Autodesk Fusion 360 part; units mm, degrees
(part 2 of 8)
  spline S4 degree 5 poles (18.7513, 10.1044) (18.7514, 10.1045) (18.7517, 10.1046) (18.7521, 10.1049) (18.7528, 10.1053) (18.7538, 10.1058) (18.755, 10.1065) (18.7564, 10.1073) (18.7579, 10.1081) (18.7595, 10.1091) (18.7613, 10.1102) (18.7633, 10.1113) (18.7654, 10.1125) (18.7676, 10.1138) (18.7699, 10.1153) (18.7724, 10.1168) (18.775, 10.1183) (18.7778, 10.12) (18.7807, 10.1218) (18.7836, 10.1236) (18.7868, 10.1256) (18.79, 10.1276) (18.7933, 10.1297) (18.7968, 10.1319) (18.8003, 10.1341) (18.804, 10.1365) (18.8078, 10.1389) (18.8117, 10.1414) (18.8157, 10.144) (18.8198, 10.1467) (18.824, 10.1495) (18.8282, 10.1523) (18.8326, 10.1553) (18.8371, 10.1583) (18.8417, 10.1613) (18.8463, 10.1645) (18.8511, 10.1677) (18.8559, 10.1711) (18.8608, 10.1745) (18.8658, 10.1779) (18.8709, 10.1815) (18.8761, 10.1851) (18.8814, 10.1888) (18.8867, 10.1926) (18.8921, 10.1965) (18.8976, 10.2004) (18.9032, 10.2044) (18.9088, 10.2085) (18.9145, 10.2127) (18.9203, 10.2169) (18.9262, 10.2212) (18.9321, 10.2256) (18.9381, 10.23) (18.9442, 10.2346) (18.9503, 10.2392) (18.9565, 10.2439) (18.9628, 10.2486) (18.9691, 10.2534) (18.9755, 10.2583) (18.982, 10.2633) (18.9885, 10.2683) (18.9951, 10.2735) (19.0017, 10.2786) (19.0085, 10.2839) (19.0152, 10.2892) (19.022, 10.2946) (19.0289, 10.3001) (19.0358, 10.3056) (19.0428, 10.3112) (19.0498, 10.3169) (19.0569, 10.3227) (19.0641, 10.3285) (19.0713, 10.3344) (19.0785, 10.3403) (19.0858, 10.3464) (19.0932, 10.3525) (19.1006, 10.3586) (19.108, 10.3649) (19.1155, 10.3712) (19.123, 10.3775) (19.1306, 10.384) (19.1382, 10.3905) (19.1459, 10.397) (19.1536, 10.4037) (19.1614, 10.4104) (19.1692, 10.4172) (19.177, 10.424) (19.1849, 10.4309) (19.1929, 10.4379) (19.2008, 10.4449) (19.2088, 10.452) (19.2169, 10.4592) (19.225, 10.4665) (19.2331, 10.4738) (19.2413, 10.4811) (19.2495, 10.4886) (19.2577, 10.4961) (19.266, 10.5036) (19.2743, 10.5113) (19.2826, 10.519) (19.291, 10.5267) (19.2994, 10.5346) (19.3079, 10.5425) (19.3163, 10.5504) (19.3249, 10.5584) (19.3334, 10.5665) (19.342, 10.5747) (19.3506, 10.5829) (19.3592, 10.5912) (19.3679, 10.5995) (19.3766, 10.6079) (19.3853, 10.6164) (19.3941, 10.6249) (19.4028, 10.6335) (19.4116, 10.6421) (19.4205, 10.6509) (19.4293, 10.6596) (19.4382, 10.6685) (19.4472, 10.6774) (19.4561, 10.6864) (19.4651, 10.6954) (19.4741, 10.7045) (19.4831, 10.7136) (19.4921, 10.7229) (19.5012, 10.7321) (19.5103, 10.7415) (19.5194, 10.7509) (19.5285, 10.7603) (19.5377, 10.7698) (19.5469, 10.7794) (19.5561, 10.7891) (19.5653, 10.7988) (19.5745, 10.8085) (19.5838, 10.8184) (19.5931, 10.8282) (19.6024, 10.8382) (19.6117, 10.8482) (19.621, 10.8583) (19.6304, 10.8684) (19.6398, 10.8786) (19.6492, 10.8888) (19.6586, 10.8991) (19.668, 10.9095) (19.6775, 10.9199) (19.6869, 10.9304) (19.6964, 10.9409) (19.7059, 10.9515) (19.7154, 10.9622) (19.725, 10.9729) (19.7345, 10.9837) (19.7441, 10.9945) (19.7536, 11.0054) (19.7632, 11.0164) (19.7728, 11.0274) (19.7824, 11.0384) (19.7921, 11.0496) (19.8017, 11.0607) (19.8113, 11.072) (19.821, 11.0833) (19.8307, 11.0946) (19.8404, 11.1061) (19.8501, 11.1175) (19.8598, 11.1291) (19.8695, 11.1406) (19.8792, 11.1523) (19.889, 11.164) (19.8987, 11.1757) (19.9085, 11.1875) (19.9183, 11.1994) (19.9281, 11.2113) (19.9379, 11.2233) (19.9477, 11.2354) (19.9575, 11.2475) (19.9673, 11.2596) (19.9771, 11.2718) (19.9869, 11.2841) (19.9968, 11.2964) (20.0066, 11.3088) (20.0165, 11.3212) (20.0263, 11.3337) (20.0362, 11.3462) (20.0461, 11.3588) (20.056, 11.3715) (20.0659, 11.3842) (20.0757, 11.3969) (20.0856, 11.4097) (20.0955, 11.4226) (20.1054, 11.4355) (20.1154, 11.4485) (20.1253, 11.4615) (20.1352, 11.4746) (20.1451, 11.4878) (20.155, 11.501) (20.165, 11.5142) (20.1749, 11.5275) (20.1848, 11.5409) (20.1948, 11.5543) (20.2047, 11.5677) (20.2147, 11.5813) (20.2246, 11.5948) (20.2346, 11.6085) (20.2445, 11.6221) (20.2545, 11.6359) (20.2644, 11.6497) (20.2744, 11.6635) (20.2843, 11.6774) (20.2943, 11.6913) (20.3042, 11.7053) (20.3142, 11.7194) (20.3242, 11.7335) (20.3341, 11.7476) (20.3441, 11.7618) (20.354, 11.7761) (20.364, 11.7904) (20.3739, 11.8048) (20.3839, 11.8192) (20.3938, 11.8336) (20.4038, 11.8482) (20.4137, 11.8627) (20.4237, 11.8773) (20.4336, 11.892) (20.4436, 11.9067) (20.4535, 11.9215) (20.4634, 11.9363) (20.4734, 11.9512) (20.4833, 11.9661) (20.4932, 11.9811) (20.5032, 11.9962) (20.5131, 12.0112) (20.523, 12.0264) (20.5329, 12.0416) (20.5428, 12.0568) (20.5527, 12.0721) (20.5626, 12.0874) (20.5725, 12.1028) (20.5824, 12.1182) (20.5923, 12.1337) (20.6022, 12.1492) (20.6121, 12.1648) (20.6219, 12.1805) (20.6318, 12.1961) (20.6397, 12.2087) (20.6456, 12.2182) (20.6495, 12.2245) (20.6515, 12.2277) knots 0 0 0 0 0 0 0.00416667 0.00833333 0.0125 0.01666667 0.02083333 0.025 0.02916667 0.03333333 0.0375 0.04166667 0.04583333 0.05 0.05416667 0.05833333 0.0625 0.06666667 0.07083333 0.075 0.07916667 0.08333333 0.0875 0.09166667 0.09583333 0.1 0.10416667 0.10833333 0.1125 0.11666667 0.12083333 0.125 0.12916667 0.13333333 0.1375 0.14166667 0.14583333 0.15 0.15416667 0.15833333 0.1625 0.16666667 0.17083333 0.175 0.17916667 0.18333333 0.1875 0.19166667 0.19583333 0.2 0.20416667 0.20833333 0.2125 0.21666667 0.22083333 0.225 0.22916667 0.23333333 0.2375 0.24166667 0.24583333 0.25 0.25416667 0.25833333 0.2625 0.26666667 0.27083333 0.275 0.27916667 0.28333333 0.2875 0.29166667 0.29583333 0.3 0.30416667 0.30833333 0.3125 0.31666667 0.32083333 0.325 0.32916667 0.33333333 0.3375 0.34166667 0.34583333 0.35 0.35416667 0.35833333 0.3625 0.36666667 0.37083333 0.375 0.37916667 0.38333333 0.3875 0.39166667 0.39583333 0.4 0.40416667 0.40833333 0.4125 0.41666667 0.42083333 0.425 0.42916667 0.43333333 0.4375 0.44166667 0.44583333 0.45 0.45416667 0.45833333 0.4625 0.46666667 0.47083333 0.475 0.47916667 0.48333333 0.4875 0.49166667 0.49583333 0.5 0.50416667 0.50833333 0.5125 0.51666667 0.52083333 0.525 0.52916667 0.53333333 0.5375 0.54166667 0.54583333 0.55 0.55416667 0.55833333 0.5625 0.56666667 0.57083333 0.575 0.57916667 0.58333333 0.5875 0.59166667 0.59583333 0.6 0.60416667 0.60833333 0.6125 0.61666667 0.62083333 0.625 0.62916667 0.63333333 0.6375 0.64166667 0.64583333 0.65 0.65416667 0.65833333 0.6625 0.66666667 0.67083333 0.675 0.67916667 0.68333333 0.6875 0.69166667 0.69583333 0.7 0.70416667 0.70833333 0.7125 0.71666667 0.72083333 0.725 0.72916667 0.73333333 0.7375 0.74166667 0.74583333 0.75 0.75416667 0.75833333 0.7625 0.76666667 0.77083333 0.775 0.77916667 0.78333333 0.7875 0.79166667 0.79583333 0.8 0.80416667 0.80833333 0.8125 0.81666667 0.82083333 0.825 0.82916667 0.83333333 0.8375 0.84166667 0.84583333 0.85 0.85416667 0.85833333 0.8625 0.86666667 0.87083333 0.875 0.87916667 0.88333333 0.8875 0.89166667 0.89583333 0.9 0.90416667 0.90833333 0.9125 0.91666667 0.92083333 0.925 0.92916667 0.93333333 0.9375 0.94166667 0.94583333 0.95 0.95416667 0.95833333 0.9625 0.96666667 0.97083333 0.975 0.97916667 0.98333333 0.9875 0.99166667 0.99583333 1 1 1 1 1 1
  arc A5 (20.6515, 12.2277) -> (19.7016, 13.7057) centre (0, 0) ccw
  spline S5 degree 5 poles (19.7016, 13.7057) (19.6979, 13.7052) (19.6905, 13.7043) (19.6795, 13.7028) (19.6647, 13.7009) (19.6464, 13.6984) (19.6281, 13.6959) (19.6098, 13.6934) (19.5916, 13.6909) (19.5734, 13.6883) (19.5552, 13.6857) (19.5371, 13.6831) (19.519, 13.6805) (19.501, 13.6778) (19.4831, 13.6752) (19.4651, 13.6724) (19.4472, 13.6697) (19.4294, 13.6669) (19.4116, 13.6642) (19.3939, 13.6614) (19.3762, 13.6585) (19.3585, 13.6557) (19.3409, 13.6528) (19.3233, 13.6499) (19.3058, 13.647) (19.2883, 13.644) (19.2709, 13.641) (19.2535, 13.638) (19.2362, 13.635) (19.2189, 13.632) (19.2016, 13.6289) (19.1844, 13.6258) (19.1673, 13.6227) (19.1502, 13.6196) (19.1331, 13.6164) (19.1161, 13.6132) (19.0991, 13.61) (19.0822, 13.6068) (19.0654, 13.6036) (19.0485, 13.6003) (19.0318, 13.597) (19.015, 13.5937) (18.9984, 13.5904) (18.9817, 13.5871) (18.9652, 13.5837) (18.9486, 13.5803) (18.9322, 13.5769) (18.9157, 13.5735) (18.8994, 13.57) (18.883, 13.5665) (18.8668, 13.563) (18.8505, 13.5595) (18.8343, 13.556) (18.8182, 13.5525) (18.8021, 13.5489) (18.7861, 13.5453) (18.7701, 13.5417) (18.7542, 13.5381) (18.7384, 13.5344) (18.7225, 13.5308) (18.7068, 13.5271) (18.6911, 13.5234) (18.6754, 13.5197) (18.6598, 13.5159) (18.6442, 13.5122) (18.6287, 13.5084) (18.6133, 13.5046) (18.5979, 13.5008) (18.5825, 13.497) (18.5672, 13.4932) (18.552, 13.4893) (18.5368, 13.4855) (18.5217, 13.4816) (18.5066, 13.4777) (18.4916, 13.4738) (18.4766, 13.4698) (18.4617, 13.4659) (18.4468, 13.4619) (18.432, 13.458) (18.4173, 13.454) (18.4026, 13.45) (18.388, 13.446) (18.3734, 13.4419) (18.3589, 13.4379) (18.3444, 13.4338) (18.33, 13.4297) (18.3157, 13.4257) (18.3014, 13.4216) (18.2871, 13.4175) (18.273, 13.4133) (18.2588, 13.4092) (18.2448, 13.405) (18.2308, 13.4009) (18.2168, 13.3967) (18.2029, 13.3925) (18.1891, 13.3883) (18.1754, 13.3841) (18.1616, 13.3799) (18.148, 13.3757) (18.1344, 13.3715) (18.1209, 13.3672) (18.1074, 13.363) (18.094, 13.3587) (18.0807, 13.3544) (18.0674, 13.3501) (18.0542, 13.3458) (18.041, 13.3415) (18.0279, 13.3372) (18.0149, 13.3329) (18.0019, 13.3286) (17.989, 13.3243) (17.9761, 13.3199) (17.9633, 13.3156) (17.9506, 13.3112) (17.938, 13.3069) (17.9254, 13.3025) (17.9128, 13.2981) (17.9004, 13.2938) (17.888, 13.2894) (17.8756, 13.285) (17.8634, 13.2806) (17.8512, 13.2762) (17.839, 13.2718) (17.827, 13.2674) (17.815, 13.263) (17.803, 13.2586) (17.7911, 13.2542) (17.7793, 13.2498) (17.7676, 13.2454) (17.7559, 13.241) (17.7443, 13.2365) (17.7328, 13.2321) (17.7213, 13.2277) (17.7099, 13.2233) (17.6986, 13.2189) (17.6874, 13.2144) (17.6762, 13.21) (17.665, 13.2056) (17.654, 13.2012) (17.643, 13.1968) (17.6321, 13.1924) (17.6213, 13.188) (17.6105, 13.1836) (17.5998, 13.1791) (17.5892, 13.1747) (17.5787, 13.1704) (17.5682, 13.166) (17.5578, 13.1616) (17.5475, 13.1572) (17.5373, 13.1528) (17.5271, 13.1484) (17.517, 13.1441) (17.507, 13.1397) (17.497, 13.1354) (17.4872, 13.131) (17.4774, 13.1267) (17.4676, 13.1224) (17.458, 13.1181) (17.4484, 13.1138) (17.439, 13.1095) (17.4296, 13.1052) (17.4202, 13.1009) (17.411, 13.0966) (17.4018, 13.0924) (17.3927, 13.0882) (17.3837, 13.0839) (17.3748, 13.0797) (17.366, 13.0755) (17.3572, 13.0714) (17.3485, 13.0672) (17.3399, 13.063) (17.3314, 13.0589) (17.323, 13.0548) (17.3146, 13.0507) (17.3064, 13.0466) (17.2982, 13.0425) (17.2901, 13.0385) (17.2821, 13.0345) (17.2742, 13.0305) (17.2664, 13.0265) (17.2586, 13.0225) (17.251, 13.0186) (17.2434, 13.0147) (17.2359, 13.0108) (17.2285, 13.0069) (17.2212, 13.0031) (17.214, 12.9993) (17.2069, 12.9955) (17.1999, 12.9918) (17.193, 12.988) (17.1861, 12.9843) (17.1794, 12.9807) (17.1728, 12.977) (17.1662, 12.9734) (17.1598, 12.9698) (17.1534, 12.9663) (17.1471, 12.9628) (17.141, 12.9593) (17.1349, 12.9559) (17.129, 12.9525) (17.1231, 12.9491) (17.1173, 12.9458) (17.1117, 12.9425) (17.1061, 12.9393) (17.1007, 12.9361) (17.0953, 12.9329) (17.0901, 12.9298) (17.085, 12.9267) (17.0799, 12.9237) (17.075, 12.9207) (17.0702, 12.9178) (17.0655, 12.9149) (17.0609, 12.9121) (17.0564, 12.9093) (17.052, 12.9066) (17.0478, 12.904) (17.0437, 12.9014) (17.0396, 12.8988) (17.0357, 12.8963) (17.0319, 12.8939) (17.0283, 12.8915) (17.0247, 12.8892) (17.0213, 12.887) (17.018, 12.8848) (17.0148, 12.8827) (17.0118, 12.8807) (17.0089, 12.8787) (17.0061, 12.8769) (17.0034, 12.8751) (17.0009, 12.8733) (16.9985, 12.8717) (16.9962, 12.8701) (16.9941, 12.8687) (16.9921, 12.8673) (16.9903, 12.866) (16.9885, 12.8648) (16.987, 12.8637) (16.9856, 12.8627) (16.9843, 12.8618) (16.9832, 12.861) (16.9823, 12.8603) (16.9816, 12.8598) (16.9812, 12.8595) (16.981, 12.8593) (16.9808, 12.8592) knots -1 -1 -1 -1 -1 -1 -0.99583333 -0.99166667 -0.9875 -0.98333333 -0.97916667 -0.975 -0.97083333 -0.96666667 -0.9625 -0.95833333 -0.95416667 -0.95 -0.94583333 -0.94166667 -0.9375 -0.93333333 -0.92916667 -0.925 -0.92083333 -0.91666667 -0.9125 -0.90833333 -0.90416667 -0.9 -0.89583333 -0.89166667 -0.8875 -0.88333333 -0.87916667 -0.875 -0.87083333 -0.86666667 -0.8625 -0.85833333 -0.85416667 -0.85 -0.84583333 -0.84166667 -0.8375 -0.83333333 -0.82916667 -0.825 -0.82083333 -0.81666667 -0.8125 -0.80833333 -0.80416667 -0.8 -0.79583333 -0.79166667 -0.7875 -0.78333333 -0.77916667 -0.775 -0.77083333 -0.76666667 -0.7625 -0.75833333 -0.75416667 -0.75 -0.74583333 -0.74166667 -0.7375 -0.73333333 -0.72916667 -0.725 -0.72083333 -0.71666667 -0.7125 -0.70833333 -0.70416667 -0.7 -0.69583333 -0.69166667 -0.6875 -0.68333333 -0.67916667 -0.675 -0.67083333 -0.66666667 -0.6625 -0.65833333 -0.65416667 -0.65 -0.64583333 -0.64166667 -0.6375 -0.63333333 -0.62916667 -0.625 -0.62083333 -0.61666667 -0.6125 -0.60833333 -0.60416667 -0.6 -0.59583333 -0.59166667 -0.5875 -0.58333333 -0.57916667 -0.575 -0.57083333 -0.56666667 -0.5625 -0.55833333 -0.55416667 -0.55 -0.54583333 -0.54166667 -0.5375 -0.53333333 -0.52916667 -0.525 -0.52083333 -0.51666667 -0.5125 -0.50833333 -0.50416667 -0.5 -0.49583333 -0.49166667 -0.4875 -0.48333333 -0.47916667 -0.475 -0.47083333 -0.46666667 -0.4625 -0.45833333 -0.45416667 -0.45 -0.44583333 -0.44166667 -0.4375 -0.43333333 -0.42916667 -0.425 -0.42083333 -0.41666667 -0.4125 -0.40833333 -0.40416667 -0.4 -0.39583333 -0.39166667 -0.3875 -0.38333333 -0.37916667 -0.375 -0.37083333 -0.36666667 -0.3625 -0.35833333 -0.35416667 -0.35 -0.34583333 -0.34166667 -0.3375 -0.33333333 -0.32916667 -0.325 -0.32083333 -0.31666667 -0.3125 -0.30833333 -0.30416667 -0.3 -0.29583333 -0.29166667 -0.2875 -0.28333333 -0.27916667 -0.275 -0.27083333 -0.26666667 -0.2625 -0.25833333 -0.25416667 -0.25 -0.24583333 -0.24166667 -0.2375 -0.23333333 -0.22916667 -0.225 -0.22083333 -0.21666667 -0.2125 -0.20833333 -0.20416667 -0.2 -0.19583333 -0.19166667 -0.1875 -0.18333333 -0.17916667 -0.175 -0.17083333 -0.16666667 -0.1625 -0.15833333 -0.15416667 -0.15 -0.14583333 -0.14166667 -0.1375 -0.13333333 -0.12916667 -0.125 -0.12083333 -0.11666667 -0.1125 -0.10833333 -0.10416667 -0.1 -0.09583333 -0.09166667 -0.0875 -0.08333333 -0.07916667 -0.075 -0.07083333 -0.06666667 -0.0625 -0.05833333 -0.05416667 -0.05 -0.04583333 -0.04166667 -0.0375 -0.03333333 -0.02916667 -0.025 -0.02083333 -0.01666667 -0.0125 -0.00833333 -0.00416667 0 0 0 0 0 0
  line L10 (16.9808, 12.8592) -> (16.9799, 12.8585)
  line L11 (16.9799, 12.8585) -> (15.5455, 11.7723)
  arc A6 (15.5455, 11.7723) -> (13.8648, 13.7119) centre (0, 0) ccw
  line L12 (13.8648, 13.7119) -> (15.1441, 14.9771)
  line L13 (15.1441, 14.9771) -> (15.145, 14.9779)
  spline S6 degree 5 poles (15.145, 14.9779) (15.1451, 14.978) (15.1453, 14.9783) (15.1456, 14.9786) (15.1462, 14.9792) (15.147, 14.98) (15.148, 14.981) (15.149, 14.9821) (15.1502, 14.9834) (15.1516, 14.9848) (15.153, 14.9863) (15.1545, 14.9879) (15.1562, 14.9897) (15.158, 14.9916) (15.1598, 14.9936) (15.1618, 14.9958) (15.1639, 14.998) (15.166, 15.0004) (15.1683, 15.0029) (15.1706, 15.0055) (15.1731, 15.0082) (15.1756, 15.0111) (15.1782, 15.014) (15.1809, 15.0171) (15.1837, 15.0203) (15.1865, 15.0236) (15.1895, 15.027) (15.1925, 15.0305) (15.1956, 15.0341) (15.1988, 15.0378) (15.202, 15.0417) (15.2053, 15.0456) (15.2087, 15.0497) (15.2121, 15.0538) (15.2157, 15.058) (15.2192, 15.0624) (15.2229, 15.0668) (15.2266, 15.0714) (15.2304, 15.076) (15.2342, 15.0808) (15.2381, 15.0856) (15.242, 15.0906) (15.246, 15.0956) (15.2501, 15.1007) (15.2542, 15.106) (15.2583, 15.1113) (15.2626, 15.1167) (15.2668, 15.1222) (15.2711, 15.1278) (15.2755, 15.1335) (15.2799, 15.1393) (15.2844, 15.1452) (15.2889, 15.1511) (15.2934, 15.1572) (15.298, 15.1634) (15.3026, 15.1696) (15.3073, 15.1759) (15.312, 15.1823) (15.3168, 15.1888) (15.3216, 15.1954) (15.3264, 15.2021) (15.3313, 15.2089) (15.3362, 15.2157) (15.3412, 15.2226) (15.3462, 15.2296) (15.3512, 15.2367) (15.3562, 15.2439) (15.3613, 15.2512) (15.3664, 15.2585) (15.3716, 15.266) (15.3768, 15.2735) (15.382, 15.2811) (15.3872, 15.2888) (15.3925, 15.2965) (15.3978, 15.3044) (15.4031, 15.3123) (15.4085, 15.3203) (15.4139, 15.3284) (15.4193, 15.3365) (15.4247, 15.3447) (15.4302, 15.3531) (15.4357, 15.3614) (15.4412, 15.3699) (15.4467, 15.3785) (15.4523, 15.3871) (15.4579, 15.3958) (15.4635, 15.4046) (15.4691, 15.4134) (15.4747, 15.4223) (15.4804, 15.4313) (15.4861, 15.4404) (15.4918, 15.4496) (15.4975, 15.4588) (15.5032, 15.4681) (15.509, 15.4775) (15.5148, 15.4869) (15.5205, 15.4964) (15.5263, 15.506) (15.5322, 15.5157) (15.538, 15.5254) (15.5439, 15.5352) (15.5497, 15.5451) (15.5556, 15.5551) (15.5615, 15.5651) (15.5674, 15.5752) (15.5733, 15.5854) (15.5793, 15.5956) (15.5852, 15.6059) (15.5912, 15.6163) (15.5971, 15.6267) (15.6031, 15.6372) (15.6091, 15.6478) (15.6151, 15.6585) (15.6211, 15.6692) (15.6271, 15.68) (15.6331, 15.6908) (15.6392, 15.7017) (15.6452, 15.7127) (15.6512, 15.7238) (15.6573, 15.7349) (15.6634, 15.7461) (15.6694, 15.7574) (15.6755, 15.7687) (15.6816, 15.7801) (15.6877, 15.7915) (15.6938, 15.803) (15.6999, 15.8146) (15.706, 15.8263) (15.7121, 15.838) (15.7182, 15.8498) (15.7243, 15.8616) (15.7304, 15.8735) (15.7365, 15.8855) (15.7426, 15.8975) (15.7487, 15.9096) (15.7549, 15.9218) (15.761, 15.934) (15.7671, 15.9463) (15.7733, 15.9587) (15.7794, 15.9711) (15.7855, 15.9836) (15.7916, 15.9961) (15.7978, 16.0087) (15.8039, 16.0214) (15.81, 16.0341) (15.8162, 16.0469) (15.8223, 16.0597) (15.8284, 16.0726) (15.8345, 16.0856) (15.8407, 16.0986) (15.8468, 16.1117) (15.8529, 16.1249) (15.859, 16.1381) (15.8651, 16.1513) (15.8712, 16.1647) (15.8773, 16.178) (15.8834, 16.1915) (15.8895, 16.205) (15.8956, 16.2186) (15.9017, 16.2322) (15.9078, 16.2459) (15.9138, 16.2596) (15.9199, 16.2734) (15.926, 16.2873) (15.932, 16.3012) (15.9381, 16.3151) (15.9441, 16.3292) (15.9502, 16.3432) (15.9562, 16.3574) (15.9622, 16.3716) (15.9683, 16.3858) (15.9743, 16.4002) (15.9803, 16.4145) (15.9863, 16.4289) (15.9923, 16.4434) (15.9982, 16.458) (16.0042, 16.4725) (16.0102, 16.4872) (16.0161, 16.5019) (16.0221, 16.5167) (16.028, 16.5315) (16.0339, 16.5463) (16.0398, 16.5613) (16.0458, 16.5762) (16.0516, 16.5913) (16.0575, 16.6063) (16.0634, 16.6215) (16.0693, 16.6367) (16.0751, 16.6519) (16.081, 16.6672) (16.0868, 16.6826) (16.0926, 16.698) (16.0984, 16.7134) (16.1042, 16.7289) (16.11, 16.7445) (16.1158, 16.7601) (16.1215, 16.7758) (16.1273, 16.7915) (16.133, 16.8073) (16.1387, 16.8231) (16.1444, 16.839) (16.1501, 16.8549) (16.1558, 16.8709) (16.1615, 16.8869) (16.1671, 16.903) (16.1728, 16.9191) (16.1784, 16.9353) (16.184, 16.9515) (16.1896, 16.9678) (16.1952, 16.9842) (16.2008, 17.0005) (16.2063, 17.017) (16.2118, 17.0335) (16.2174, 17.05) (16.2229, 17.0666) (16.2284, 17.0832) (16.2338, 17.0999) (16.2393, 17.1166) (16.2447, 17.1334) (16.2501, 17.1502) (16.2556, 17.1671) (16.2609, 17.1841) (16.2663, 17.201) (16.2717, 17.2181) (16.277, 17.2351) (16.2823, 17.2522) (16.2876, 17.2694) (16.2929, 17.2866) (16.2982, 17.3039) (16.3035, 17.3212) (16.3087, 17.3386) (16.3139, 17.356) (16.3191, 17.3734) (16.3243, 17.3909) (16.3294, 17.4085) (16.3346, 17.4261) (16.3397, 17.4437) (16.3448, 17.4614) (16.3499, 17.4791) (16.355, 17.4969) (16.36, 17.5148) (16.364, 17.529) (16.367, 17.5398) (16.369, 17.547) (16.37, 17.5506) knots 0 0 0 0 0 0 0.00416667 0.00833333 0.0125 0.01666667 0.02083333 0.025 0.02916667 0.03333333 0.0375 0.04166667 0.04583333 0.05 0.05416667 0.05833333 0.0625 0.06666667 0.07083333 0.075 0.07916667 0.08333333 0.0875 0.09166667 0.09583333 0.1 0.10416667 0.10833333 0.1125 0.11666667 0.12083333 0.125 0.12916667 0.13333333 0.1375 0.14166667 0.14583333 0.15 0.15416667 0.15833333 0.1625 0.16666667 0.17083333 0.175 0.17916667 0.18333333 0.1875 0.19166667 0.19583333 0.2 0.20416667 0.20833333 0.2125 0.21666667 0.22083333 0.225 0.22916667 0.23333333 0.2375 0.24166667 0.24583333 0.25 0.25416667 0.25833333 0.2625 0.26666667 0.27083333 0.275 0.27916667 0.28333333 0.2875 0.29166667 0.29583333 0.3 0.30416667 0.30833333 0.3125 0.31666667 0.32083333 0.325 0.32916667 0.33333333 0.3375 0.34166667 0.34583333 0.35 0.35416667 0.35833333 0.3625 0.36666667 0.37083333 0.375 0.37916667 0.38333333 0.3875 0.39166667 0.39583333 0.4 0.40416667 0.40833333 0.4125 0.41666667 0.42083333 0.425 0.42916667 0.43333333 0.4375 0.44166667 0.44583333 0.45 0.45416667 0.45833333 0.4625 0.46666667 0.47083333 0.475 0.47916667 0.48333333 0.4875 0.49166667 0.49583333 0.5 0.50416667 0.50833333 0.5125 0.51666667 0.52083333 0.525 0.52916667 0.53333333 0.5375 0.54166667 0.54583333 0.55 0.55416667 0.55833333 0.5625 0.56666667 0.57083333 0.575 0.57916667 0.58333333 0.5875 0.59166667 0.59583333 0.6 0.60416667 0.60833333 0.6125 0.61666667 0.62083333 0.625 0.62916667 0.63333333 0.6375 0.64166667 0.64583333 0.65 0.65416667 0.65833333 0.6625 0.66666667 0.67083333 0.675 0.67916667 0.68333333 0.6875 0.69166667 0.69583333 0.7 0.70416667 0.70833333 0.7125 0.71666667 0.72083333 0.725 0.72916667 0.73333333 0.7375 0.74166667 0.74583333 0.75 0.75416667 0.75833333 0.7625 0.76666667 0.77083333 0.775 0.77916667 0.78333333 0.7875 0.79166667 0.79583333 0.8 0.80416667 0.80833333 0.8125 0.81666667 0.82083333 0.825 0.82916667 0.83333333 0.8375 0.84166667 0.84583333 0.85 0.85416667 0.85833333 0.8625 0.86666667 0.87083333 0.875 0.87916667 0.88333333 0.8875 0.89166667 0.89583333 0.9 0.90416667 0.90833333 0.9125 0.91666667 0.92083333 0.925 0.92916667 0.93333333 0.9375 0.94166667 0.94583333 0.95 0.95416667 0.95833333 0.9625 0.96666667 0.97083333 0.975 0.97916667 0.98333333 0.9875 0.99166667 0.99583333 1 1 1 1 1 1
  arc A7 (16.37, 17.5506) -> (15.0422, 18.7011) centre (0, 0) ccw
  spline S7 degree 5 poles (15.0422, 18.7011) (15.0388, 18.6996) (15.032, 18.6966) (15.0218, 18.6921) (15.0082, 18.6861) (14.9913, 18.6786) (14.9744, 18.671) (14.9576, 18.6635) (14.9408, 18.6559) (14.9241, 18.6483) (14.9074, 18.6407) (14.8907, 18.6331) (14.8741, 18.6255) (14.8576, 18.6179) (14.8411, 18.6102) (14.8247, 18.6026) (14.8083, 18.5949) (14.792, 18.5872) (14.7757, 18.5796) (14.7594, 18.5719) (14.7432, 18.5642) (14.7271, 18.5564) (14.711, 18.5487) (14.695, 18.541) (14.679, 18.5332) (14.663, 18.5255) (14.6472, 18.5177) (14.6313, 18.5099) (14.6155, 18.5022) (14.5998, 18.4944) (14.5841, 18.4866) (14.5685, 18.4788) (14.5529, 18.4709) (14.5374, 18.4631) (14.5219, 18.4553) (14.5065, 18.4474) (14.4911, 18.4396) (14.4758, 18.4317) (14.4605, 18.4239) (14.4453, 18.416) (14.4301, 18.4081) (14.415, 18.4002) (14.3999, 18.3924) (14.3849, 18.3845) (14.37, 18.3766) (14.3551, 18.3686) (14.3402, 18.3607) (14.3254, 18.3528) (14.3107, 18.3449) (14.296, 18.337) (14.2814, 18.329) (14.2668, 18.3211) (14.2523, 18.3131) (14.2378, 18.3052) (14.2234, 18.2972) (14.209, 18.2893) (14.1947, 18.2813) (14.1804, 18.2734) (14.1662, 18.2654) (14.1521, 18.2574) (14.138, 18.2494) (14.124, 18.2415) (14.11, 18.2335) (14.096, 18.2255) (14.0822, 18.2175) (14.0684, 18.2096) (14.0546, 18.2016) (14.0409, 18.1936) (14.0272, 18.1856) (14.0137, 18.1776) (14.0001, 18.1696) (13.9866, 18.1616) (13.9732, 18.1536) (13.9598, 18.1457) (13.9465, 18.1377) (13.9333, 18.1297) (13.9201, 18.1217) (13.907, 18.1137) (13.8939, 18.1057) (13.8808, 18.0978) (13.8679, 18.0898) (13.855, 18.0818) (13.8421, 18.0738) (13.8293, 18.0658) (13.8166, 18.0579) (13.8039, 18.0499) (13.7913, 18.0419) (13.7787, 18.034) (13.7662, 18.026) (13.7538, 18.0181) (13.7414, 18.0101) (13.7291, 18.0022) (13.7168, 17.9943) (13.7046, 17.9863) (13.6925, 17.9784) (13.6804, 17.9705) (13.6684, 17.9626) (13.6564, 17.9547) (13.6445, 17.9468) (13.6327, 17.9389) (13.6209, 17.931) (13.6092, 17.9231) (13.5975, 17.9152) (13.5859, 17.9074) (13.5744, 17.8995) (13.5629, 17.8917) (13.5515, 17.8839) (13.5401, 17.876) (13.5288, 17.8682) (13.5176, 17.8604) (13.5064, 17.8526) (13.4953, 17.8448) (13.4843, 17.8371) (13.4733, 17.8293) (13.4624, 17.8216) (13.4515, 17.8138) (13.4407, 17.8061) (13.43, 17.7984) (13.4193, 17.7907) (13.4087, 17.783) (13.3982, 17.7754) (13.3877, 17.7677) (13.3773, 17.7601) (13.367, 17.7524) (13.3567, 17.7448) (13.3465, 17.7372) (13.3363, 17.7297) (13.3262, 17.7221) (13.3162, 17.7146) (13.3063, 17.707) (13.2964, 17.6995) (13.2866, 17.692) (13.2768, 17.6846) (13.2671, 17.6771) (13.2575, 17.6697) (13.2479, 17.6623) (13.2385, 17.6549) (13.229, 17.6475) (13.2197, 17.6402) (13.2104, 17.6328) (13.2012, 17.6255) (13.192, 17.6182) (13.1829, 17.611) (13.1739, 17.6037) (13.165, 17.5965) (13.1561, 17.5893) (13.1473, 17.5822) (13.1386, 17.575) (13.1299, 17.5679) (13.1213, 17.5609) (13.1128, 17.5538) (13.1043, 17.5468) (13.0959, 17.5398) (13.0876, 17.5328) (13.0794, 17.5258) (13.0712, 17.5189) (13.0631, 17.512) (13.055, 17.5052) (13.0471, 17.4984) (13.0392, 17.4916) (13.0314, 17.4848) (13.0236, 17.4781) (13.016, 17.4714) (13.0084, 17.4647) (13.0008, 17.4581) (12.9934, 17.4515) (12.986, 17.445) (12.9787, 17.4384) (12.9715, 17.432) (12.9643, 17.4255) (12.9572, 17.4191) (12.9502, 17.4127) (12.9433, 17.4064) (12.9365, 17.4001) (12.9297, 17.3939) (12.923, 17.3877) (12.9164, 17.3815) (12.9098, 17.3754) (12.9033, 17.3694) (12.897, 17.3633) (12.8906, 17.3574) (12.8844, 17.3514) (12.8783, 17.3455) (12.8722, 17.3397) (12.8662, 17.3339) (12.8603, 17.3282) (12.8544, 17.3225) (12.8487, 17.3168) (12.843, 17.3113) (12.8374, 17.3057) (12.8319, 17.3003) (12.8264, 17.2948) (12.8211, 17.2895) (12.8158, 17.2842) (12.8106, 17.2789) (12.8055, 17.2737) (12.8005, 17.2686) (12.7956, 17.2635) (12.7908, 17.2585) (12.786, 17.2536) (12.7813, 17.2487) (12.7767, 17.2439) (12.7722, 17.2392) (12.7678, 17.2345) (12.7635, 17.2299) (12.7592, 17.2253) (12.7551, 17.2209) (12.751, 17.2165) (12.747, 17.2122) (12.7432, 17.2079) (12.7394, 17.2038) (12.7357, 17.1997) (12.732, 17.1957) (12.7285, 17.1918) (12.7251, 17.1879) (12.7218, 17.1842) (12.7185, 17.1805) (12.7154, 17.1769) (12.7124, 17.1734) (12.7094, 17.17) (12.7065, 17.1667) (12.7038, 17.1635) (12.7011, 17.1604) (12.6986, 17.1574) (12.6961, 17.1545) (12.6938, 17.1517) (12.6915, 17.149) (12.6894, 17.1464) (12.6873, 17.1439) (12.6854, 17.1416) (12.6835, 17.1393) (12.6818, 17.1372) (12.6802, 17.1352) (12.6787, 17.1333) (12.6773, 17.1315) (12.676, 17.1299) (12.6748, 17.1284) (12.6737, 17.127) (12.6728, 17.1258) (12.6719, 17.1247) (12.6712, 17.1238) (12.6707, 17.1232) (12.6704, 17.1228) (12.6702, 17.1225) (12.6701, 17.1224) knots -1 -1 -1 -1 -1 -1 -0.99583333 -0.99166667 -0.9875 -0.98333333 -0.97916667 -0.975 -0.97083333 -0.96666667 -0.9625 -0.95833333 -0.95416667 -0.95 -0.94583333 -0.94166667 -0.9375 -0.93333333 -0.92916667 -0.925 -0.92083333 -0.91666667 -0.9125 -0.90833333 -0.90416667 -0.9 -0.89583333 -0.89166667 -0.8875 -0.88333333 -0.87916667 -0.875 -0.87083333 -0.86666667 -0.8625 -0.85833333 -0.85416667 -0.85 -0.84583333 -0.84166667 -0.8375 -0.83333333 -0.82916667 -0.825 -0.82083333 -0.81666667 -0.8125 -0.80833333 -0.80416667 -0.8 -0.79583333 -0.79166667 -0.7875 -0.78333333 -0.77916667 -0.775 -0.77083333 -0.76666667 -0.7625 -0.75833333 -0.75416667 -0.75 -0.74583333 -0.74166667 -0.7375 -0.73333333 -0.72916667 -0.725 -0.72083333 -0.71666667 -0.7125 -0.70833333 -0.70416667 -0.7 -0.69583333 -0.69166667 -0.6875 -0.68333333 -0.67916667 -0.675 -0.67083333 -0.66666667 -0.6625 -0.65833333 -0.65416667 -0.65 -0.64583333 -0.64166667 -0.6375 -0.63333333 -0.62916667 -0.625 -0.62083333 -0.61666667 -0.6125 -0.60833333 -0.60416667 -0.6 -0.59583333 -0.59166667 -0.5875 -0.58333333 -0.57916667 -0.575 -0.57083333 -0.56666667 -0.5625 -0.55833333 -0.55416667 -0.55 -0.54583333 -0.54166667 -0.5375 -0.53333333 -0.52916667 -0.525 -0.52083333 -0.51666667 -0.5125 -0.50833333 -0.50416667 -0.5 -0.49583333 -0.49166667 -0.4875 -0.48333333 -0.47916667 -0.475 -0.47083333 -0.46666667 -0.4625 -0.45833333 -0.45416667 -0.45 -0.44583333 -0.44166667 -0.4375 -0.43333333 -0.42916667 -0.425 -0.42083333 -0.41666667 -0.4125 -0.40833333 -0.40416667 -0.4 -0.39583333 -0.39166667 -0.3875 -0.38333333 -0.37916667 -0.375 -0.37083333 -0.36666667 -0.3625 -0.35833333 -0.35416667 -0.35 -0.34583333 -0.34166667 -0.3375 -0.33333333 -0.32916667 -0.325 -0.32083333 -0.31666667 -0.3125 -0.30833333 -0.30416667 -0.3 -0.29583333 -0.29166667 -0.2875 -0.28333333 -0.27916667 -0.275 -0.27083333 -0.26666667 -0.2625 -0.25833333 -0.25416667 -0.25 -0.24583333 -0.24166667 -0.2375 -0.23333333 -0.22916667 -0.225 -0.22083333 -0.21666667 -0.2125 -0.20833333 -0.20416667 -0.2 -0.19583333 -0.19166667 -0.1875 -0.18333333 -0.17916667 -0.175 -0.17083333 -0.16666667 -0.1625 -0.15833333 -0.15416667 -0.15 -0.14583333 -0.14166667 -0.1375 -0.13333333 -0.12916667 -0.125 -0.12083333 -0.11666667 -0.1125 -0.10833333 -0.10416667 -0.1 -0.09583333 -0.09166667 -0.0875 -0.08333333 -0.07916667 -0.075 -0.07083333 -0.06666667 -0.0625 -0.05833333 -0.05416667 -0.05 -0.04583333 -0.04166667 -0.0375 -0.03333333 -0.02916667 -0.025 -0.02083333 -0.01666667 -0.0125 -0.00833333 -0.00416667 0 0 0 0 0 0
  line L14 (12.6701, 17.1224) -> (12.6694, 17.1214)
  line L15 (12.6694, 17.1214) -> (11.5992, 15.6751)
  arc A8 (11.5992, 15.6751) -> (9.4401, 17.0627) centre (0, 0) ccw
  line L16 (9.4401, 17.0627) -> (10.3111, 18.637)
  line L17 (10.3111, 18.637) -> (10.3117, 18.6381)
  spline S8 degree 5 poles (10.3117, 18.6381) (10.3118, 18.6382) (10.3119, 18.6385) (10.3122, 18.6389) (10.3125, 18.6396) (10.3131, 18.6406) (10.3137, 18.6419) (10.3144, 18.6432) (10.3152, 18.6448) (10.3161, 18.6465) (10.3171, 18.6483) (10.3181, 18.6503) (10.3192, 18.6525) (10.3203, 18.6548) (10.3216, 18.6573) (10.3228, 18.6599) (10.3242, 18.6626) (10.3256, 18.6655) (10.327, 18.6686) (10.3286, 18.6717) (10.3301, 18.675) (10.3318, 18.6785) (10.3334, 18.6821) (10.3352, 18.6858) (10.3369, 18.6896) (10.3388, 18.6936) (10.3406, 18.6977) (10.3425, 18.7019) (10.3445, 18.7062) (10.3465, 18.7107) (10.3485, 18.7153) (10.3506, 18.72) (10.3527, 18.7248) (10.3548, 18.7298) (10.357, 18.7348) (10.3592, 18.74) (10.3614, 18.7453) (10.3637, 18.7507) (10.366, 18.7562) (10.3683, 18.7619) (10.3707, 18.7676) (10.3731, 18.7735) (10.3755, 18.7794) (10.378, 18.7855) (10.3804, 18.7917) (10.3829, 18.7979) (10.3854, 18.8043) (10.388, 18.8108) (10.3905, 18.8174) (10.3931, 18.8241) (10.3957, 18.8309) (10.3983, 18.8378) (10.401, 18.8448) (10.4036, 18.8519) (10.4063, 18.8591) (10.409, 18.8664) (10.4117, 18.8738) (10.4144, 18.8812) (10.4172, 18.8888) (10.4199, 18.8965) (10.4227, 18.9043) (10.4254, 18.9121) (10.4282, 18.9201) (10.431, 18.9281) (10.4338, 18.9362) (10.4367, 18.9445) (10.4395, 18.9528) (10.4423, 18.9612) (10.4452, 18.9697) (10.448, 18.9783) (10.4509, 18.9869) (10.4537, 18.9957) (10.4566, 19.0045) (10.4595, 19.0135) (10.4623, 19.0225) (10.4652, 19.0316) (10.4681, 19.0408) (10.471, 19.05) (10.4739, 19.0594) (10.4768, 19.0688) (10.4797, 19.0783) (10.4826, 19.0879) (10.4855, 19.0976) (10.4884, 19.1074) (10.4913, 19.1172) (10.4942, 19.1271) (10.4971, 19.1371) (10.5, 19.1472) (10.5029, 19.1574) (10.5058, 19.1676) (10.5087, 19.1779) (10.5116, 19.1883) (10.5145, 19.1988) (10.5174, 19.2093) (10.5202, 19.2199) (10.5231, 19.2306) (10.526, 19.2414) (10.5289, 19.2522) (10.5317, 19.2631) (10.5346, 19.2741) (10.5374, 19.2852) (10.5403, 19.2963) (10.5431, 19.3075) (10.546, 19.3188) (10.5488, 19.3301) (10.5516, 19.3415) (10.5544, 19.353) (10.5572, 19.3646) (10.56, 19.3762) (10.5628, 19.3879) (10.5655, 19.3997) (10.5683, 19.4115) (10.5711, 19.4234) (10.5738, 19.4354) (10.5765, 19.4475) (10.5793, 19.4596) (10.582, 19.4718) (10.5847, 19.484) (10.5874, 19.4963) (10.59, 19.5087) (10.5927, 19.5211) (10.5953, 19.5337) (10.598, 19.5462) (10.6006, 19.5589) (10.6032, 19.5716) (10.6058, 19.5843) (10.6084, 19.5972) (10.611, 19.6101) (10.6135, 19.623) (10.6161, 19.6361) (10.6186, 19.6492) (10.6211, 19.6623) (10.6236, 19.6755) (10.6261, 19.6888) (10.6286, 19.7021) (10.631, 19.7155) (10.6334, 19.729) (10.6359, 19.7425) (10.6383, 19.7561) (10.6406, 19.7697) (10.643, 19.7834) (10.6453, 19.7972) (10.6477, 19.811) (10.65, 19.8249) (10.6523, 19.8388) (10.6546, 19.8528) (10.6568, 19.8668) (10.6591, 19.8809) (10.6613, 19.8951) (10.6635, 19.9093) (10.6657, 19.9236) (10.6678, 19.938) (10.67, 19.9524) (10.6721, 19.9668) (10.6742, 19.9813) (10.6763, 19.9959) (10.6784, 20.0105) (10.6804, 20.0252) (10.6824, 20.0399) (10.6844, 20.0547) (10.6864, 20.0695) (10.6884, 20.0844) (10.6903, 20.0994) (10.6922, 20.1144) (10.6941, 20.1294) (10.696, 20.1445) (10.6978, 20.1597) (10.6997, 20.1749) (10.7015, 20.1902) (10.7032, 20.2055) (10.705, 20.2209) (10.7067, 20.2363) (10.7085, 20.2518) (10.7101, 20.2673) (10.7118, 20.2829) (10.7135, 20.2985) (10.7151, 20.3142) (10.7167, 20.3299) (10.7182, 20.3457) (10.7198, 20.3616) (10.7213, 20.3774) (10.7228, 20.3934) (10.7243, 20.4094) (10.7257, 20.4254) (10.7271, 20.4415) (10.7285, 20.4576) (10.7299, 20.4738) (10.7313, 20.49) (10.7326, 20.5063) (10.7339, 20.5226) (10.7352, 20.539) (10.7364, 20.5554) (10.7376, 20.5719) (10.7388, 20.5884) (10.74, 20.6049) (10.7411, 20.6215) (10.7422, 20.6382) (10.7433, 20.6549) (10.7444, 20.6717) (10.7454, 20.6885) (10.7464, 20.7053) (10.7474, 20.7222) (10.7483, 20.7391) (10.7492, 20.7561) (10.7501, 20.7731) (10.751, 20.7902) (10.7518, 20.8073) (10.7526, 20.8244) (10.7534, 20.8416) (10.7542, 20.8589) (10.7549, 20.8762) (10.7556, 20.8935) (10.7563, 20.9109) (10.7569, 20.9283) (10.7575, 20.9458) (10.7581, 20.9633) (10.7586, 20.9808) (10.7592, 20.9984) (10.7597, 21.0161) (10.7601, 21.0337) (10.7606, 21.0515) (10.761, 21.0692) (10.7613, 21.087) (10.7617, 21.1049) (10.762, 21.1227) (10.7623, 21.1407) (10.7625, 21.1586) (10.7627, 21.1767) (10.7629, 21.1947) (10.7631, 21.2128) (10.7632, 21.2309) (10.7633, 21.2491) (10.7634, 21.2673) (10.7634, 21.2856) (10.7634, 21.3039) (10.7634, 21.3222) (10.7634, 21.3406) (10.7633, 21.359) (10.7632, 21.3774) (10.763, 21.3959) (10.7628, 21.4144) (10.7627, 21.4293) (10.7625, 21.4404) (10.7624, 21.4479) (10.7624, 21.4516) knots 0 0 0 0 0 0 0.00416667 0.00833333 0.0125 0.01666667 0.02083333 0.025 0.02916667 0.03333333 0.0375 0.04166667 0.04583333 0.05 0.05416667 0.05833333 0.0625 0.06666667 0.07083333 0.075 0.07916667 0.08333333 0.0875 0.09166667 0.09583333 0.1 0.10416667 0.10833333 0.1125 0.11666667 0.12083333 0.125 0.12916667 0.13333333 0.1375 0.14166667 0.14583333 0.15 0.15416667 0.15833333 0.1625 0.16666667 0.17083333 0.175 0.17916667 0.18333333 0.1875 0.19166667 0.19583333 0.2 0.20416667 0.20833333 0.2125 0.21666667 0.22083333 0.225 0.22916667 0.23333333 0.2375 0.24166667 0.24583333 0.25 0.25416667 0.25833333 0.2625 0.26666667 0.27083333 0.275 0.27916667 0.28333333 0.2875 0.29166667 0.29583333 0.3 0.30416667 0.30833333 0.3125 0.31666667 0.32083333 0.325 0.32916667 0.33333333 0.3375 0.34166667 0.34583333 0.35 0.35416667 0.35833333 0.3625 0.36666667 0.37083333 0.375 0.37916667 0.38333333 0.3875 0.39166667 0.39583333 0.4 0.40416667 0.40833333 0.4125 0.41666667 0.42083333 0.425 0.42916667 0.43333333 0.4375 0.44166667 0.44583333 0.45 0.45416667 0.45833333 0.4625 0.46666667 0.47083333 0.475 0.47916667 0.48333333 0.4875 0.49166667 0.49583333 0.5 0.50416667 0.50833333 0.5125 0.51666667 0.52083333 0.525 0.52916667 0.53333333 0.5375 0.54166667 0.54583333 0.55 0.55416667 0.55833333 0.5625 0.56666667 0.57083333 0.575 0.57916667 0.58333333 0.5875 0.59166667 0.59583333 0.6 0.60416667 0.60833333 0.6125 0.61666667 0.62083333 0.625 0.62916667 0.63333333 0.6375 0.64166667 0.64583333 0.65 0.65416667 0.65833333 0.6625 0.66666667 0.67083333 0.675 0.67916667 0.68333333 0.6875 0.69166667 0.69583333 0.7 0.70416667 0.70833333 0.7125 0.71666667 0.72083333 0.725 0.72916667 0.73333333 0.7375 0.74166667 0.74583333 0.75 0.75416667 0.75833333 0.7625 0.76666667 0.77083333 0.775 0.77916667 0.78333333 0.7875 0.79166667 0.79583333 0.8 0.80416667 0.80833333 0.8125 0.81666667 0.82083333 0.825 0.82916667 0.83333333 0.8375 0.84166667 0.84583333 0.85 0.85416667 0.85833333 0.8625 0.86666667 0.87083333 0.875 0.87916667 0.88333333 0.8875 0.89166667 0.89583333 0.9 0.90416667 0.90833333 0.9125 0.91666667 0.92083333 0.925 0.92916667 0.93333333 0.9375 0.94166667 0.94583333 0.95 0.95416667 0.95833333 0.9625 0.96666667 0.97083333 0.975 0.97916667 0.98333333 0.9875 0.99166667 0.99583333 1 1 1 1 1 1
  arc A9 (10.7624, 21.4516) -> (9.1642, 22.1815) centre (0, 0) ccw
  spline S9 degree 5 poles (9.1642, 22.1815) (9.1613, 22.1791) (9.1556, 22.1743) (9.1471, 22.1671) (9.1358, 22.1575) (9.1217, 22.1455) (9.1076, 22.1335) (9.0936, 22.1215) (9.0796, 22.1095) (9.0657, 22.0975) (9.0518, 22.0855) (9.038, 22.0735) (9.0242, 22.0616) (9.0105, 22.0496) (8.9968, 22.0376) (8.9832, 22.0256) (8.9697, 22.0137) (8.9561, 22.0017) (8.9427, 21.9897) (8.9293, 21.9778) (8.9159, 21.9658) (8.9026, 21.9539) (8.8893, 21.9419) (8.8761, 21.93) (8.863, 21.9181) (8.8499, 21.9061) (8.8368, 21.8942) (8.8238, 21.8823) (8.8108, 21.8704) (8.7979, 21.8585) (8.7851, 21.8465) (8.7723, 21.8347) (8.7595, 21.8228) (8.7468, 21.8109) (8.7342, 21.799) (8.7216, 21.7871) (8.7091, 21.7753) (8.6966, 21.7634) (8.6841, 21.7516) (8.6718, 21.7397) (8.6594, 21.7279) (8.6471, 21.7161) (8.6349, 21.7043) (8.6227, 21.6925) (8.6106, 21.6807) (8.5986, 21.6689) (8.5865, 21.6571) (8.5746, 21.6453) (8.5627, 21.6336) (8.5508, 21.6218) (8.539, 21.6101) (8.5272, 21.5984) (8.5155, 21.5867) (8.5039, 21.5749) (8.4923, 21.5633) (8.4808, 21.5516) (8.4693, 21.5399) (8.4578, 21.5282) (8.4464, 21.5166) (8.4351, 21.505) (8.4238, 21.4934) (8.4126, 21.4817) (8.4014, 21.4702) (8.3903, 21.4586) (8.3793, 21.447) (8.3683, 21.4355) (8.3573, 21.4239) (8.3464, 21.4124) (8.3356, 21.4009) (8.3248, 21.3894) (8.314, 21.3779) (8.3034, 21.3665) (8.2927, 21.355) (8.2822, 21.3436) (8.2716, 21.3322) (8.2612, 21.3208) (8.2508, 21.3094) (8.2404, 21.298) (8.2301, 21.2867) (8.2198, 21.2754) (8.2097, 21.264) (8.1995, 21.2527) (8.1894, 21.2415) (8.1794, 21.2302) (8.1694, 21.219) (8.1595, 21.2078) (8.1497, 21.1966) (8.1398, 21.1854) (8.1301, 21.1743) (8.1204, 21.1631) (8.1108, 21.152) (8.1012, 21.1409) (8.0916, 21.1298) (8.0822, 21.1188) (8.0727, 21.1078) (8.0634, 21.0968) (8.0541, 21.0858) (8.0448, 21.0748) (8.0356, 21.0639) (8.0265, 21.053) (8.0174, 21.0421) (8.0084, 21.0312) (7.9994, 21.0204) (7.9905, 21.0096) (7.9816, 20.9988) (7.9728, 20.9881) (7.9641, 20.9773) (7.9554, 20.9666) (7.9467, 20.9559) (7.9382, 20.9453) (7.9296, 20.9347) (7.9212, 20.9241) (7.9128, 20.9135) (7.9044, 20.903) (7.8961, 20.8925) (7.8879, 20.882) (7.8797, 20.8715) (7.8716, 20.8611) (7.8635, 20.8507) (7.8555, 20.8404) (7.8476, 20.83) (7.8397, 20.8197) (7.8319, 20.8095) (7.8241, 20.7993) (7.8164, 20.7891) (7.8087, 20.7789) (7.8011, 20.7688) (7.7935, 20.7587) (7.7861, 20.7486) (7.7786, 20.7386) (7.7713, 20.7286) (7.7639, 20.7186) (7.7567, 20.7087) (7.7495, 20.6988) (7.7424, 20.689) (7.7353, 20.6792) (7.7283, 20.6694) (7.7213, 20.6597) (7.7144, 20.65) (7.7075, 20.6404) (7.7008, 20.6308) (7.694, 20.6212) (7.6874, 20.6117) (7.6807, 20.6022) (7.6742, 20.5928) (7.6677, 20.5834) (7.6613, 20.574) (7.6549, 20.5647) (7.6486, 20.5554) (7.6423, 20.5462) (7.6361, 20.537) (7.63, 20.5279) (7.6239, 20.5188) (7.6179, 20.5098) (7.612, 20.5008) (7.6061, 20.4919) (7.6002, 20.483) (7.5944, 20.4741) (7.5887, 20.4653) (7.5831, 20.4566) (7.5775, 20.4479) (7.5719, 20.4393) (7.5665, 20.4307) (7.5611, 20.4222) (7.5557, 20.4137) (7.5504, 20.4053) (7.5452, 20.3969) (7.54, 20.3886) (7.5349, 20.3803) (7.5298, 20.3721) (7.5249, 20.364) (7.5199, 20.3559) (7.5151, 20.3479) (7.5103, 20.3399) (7.5055, 20.332) (7.5008, 20.3242) (7.4962, 20.3164) (7.4917, 20.3087) (7.4872, 20.3011) (7.4827, 20.2935) (7.4784, 20.286) (7.474, 20.2785) (7.4698, 20.2711) (7.4656, 20.2638) (7.4615, 20.2566) (7.4574, 20.2494) (7.4534, 20.2423) (7.4495, 20.2353) (7.4456, 20.2283) (7.4418, 20.2214) (7.4381, 20.2146) (7.4344, 20.2079) (7.4307, 20.2013) (7.4272, 20.1947) (7.4237, 20.1882) (7.4203, 20.1818) (7.4169, 20.1754) (7.4136, 20.1692) (7.4103, 20.163) (7.4072, 20.1569) (7.4041, 20.1509) (7.401, 20.145) (7.398, 20.1392) (7.3951, 20.1335) (7.3922, 20.1278) (7.3895, 20.1223) (7.3867, 20.1168) (7.3841, 20.1115) (7.3815, 20.1062) (7.3789, 20.1011) (7.3765, 20.096) (7.3741, 20.091) (7.3717, 20.0862) (7.3695, 20.0814) (7.3673, 20.0768) (7.3651, 20.0722) (7.363, 20.0678) (7.361, 20.0635) (7.3591, 20.0593) (7.3572, 20.0552) (7.3554, 20.0512) (7.3537, 20.0474) (7.352, 20.0436) (7.3504, 20.04) (7.3489, 20.0366) (7.3474, 20.0332) (7.346, 20.03) (7.3446, 20.0269) (7.3434, 20.0239) (7.3422, 20.0211) (7.3411, 20.0184) (7.34, 20.0159) (7.339, 20.0135) (7.3381, 20.0113) (7.3372, 20.0092) (7.3364, 20.0073) (7.3357, 20.0055) (7.3351, 20.0039) (7.3345, 20.0024) (7.334, 20.0011) (7.3336, 20) (7.3333, 19.9993) (7.3331, 19.9988) (7.333, 19.9985) (7.333, 19.9984) knots -1 -1 -1 -1 -1 -1 -0.99583333 -0.99166667 -0.9875 -0.98333333 -0.97916667 -0.975 -0.97083333 -0.96666667 -0.9625 -0.95833333 -0.95416667 -0.95 -0.94583333 -0.94166667 -0.9375 -0.93333333 -0.92916667 -0.925 -0.92083333 -0.91666667 -0.9125 -0.90833333 -0.90416667 -0.9 -0.89583333 -0.89166667 -0.8875 -0.88333333 -0.87916667 -0.875 -0.87083333 -0.86666667 -0.8625 -0.85833333 -0.85416667 -0.85 -0.84583333 -0.84166667 -0.8375 -0.83333333 -0.82916667 -0.825 -0.82083333 -0.81666667 -0.8125 -0.80833333 -0.80416667 -0.8 -0.79583333 -0.79166667 -0.7875 -0.78333333 -0.77916667 -0.775 -0.77083333 -0.76666667 -0.7625 -0.75833333 -0.75416667 -0.75 -0.74583333 -0.74166667 -0.7375 -0.73333333 -0.72916667 -0.725 -0.72083333 -0.71666667 -0.7125 -0.70833333 -0.70416667 -0.7 -0.69583333 -0.69166667 -0.6875 -0.68333333 -0.67916667 -0.675 -0.67083333 -0.66666667 -0.6625 -0.65833333 -0.65416667 -0.65 -0.64583333 -0.64166667 -0.6375 -0.63333333 -0.62916667 -0.625 -0.62083333 -0.61666667 -0.6125 -0.60833333 -0.60416667 -0.6 -0.59583333 -0.59166667 -0.5875 -0.58333333 -0.57916667 -0.575 -0.57083333 -0.56666667 -0.5625 -0.55833333 -0.55416667 -0.55 -0.54583333 -0.54166667 -0.5375 -0.53333333 -0.52916667 -0.525 -0.52083333 -0.51666667 -0.5125 -0.50833333 -0.50416667 -0.5 -0.49583333 -0.49166667 -0.4875 -0.48333333 -0.47916667 -0.475 -0.47083333 -0.46666667 -0.4625 -0.45833333 -0.45416667 -0.45 -0.44583333 -0.44166667 -0.4375 -0.43333333 -0.42916667 -0.425 -0.42083333 -0.41666667 -0.4125 -0.40833333 -0.40416667 -0.4 -0.39583333 -0.39166667 -0.3875 -0.38333333 -0.37916667 -0.375 -0.37083333 -0.36666667 -0.3625 -0.35833333 -0.35416667 -0.35 -0.34583333 -0.34166667 -0.3375 -0.33333333 -0.32916667 -0.325 -0.32083333 -0.31666667 -0.3125 -0.30833333 -0.30416667 -0.3 -0.29583333 -0.29166667 -0.2875 -0.28333333 -0.27916667 -0.275 -0.27083333 -0.26666667 -0.2625 -0.25833333 -0.25416667 -0.25 -0.24583333 -0.24166667 -0.2375 -0.23333333 -0.22916667 -0.225 -0.22083333 -0.21666667 -0.2125 -0.20833333 -0.20416667 -0.2 -0.19583333 -0.19166667 -0.1875 -0.18333333 -0.17916667 -0.175 -0.17083333 -0.16666667 -0.1625 -0.15833333 -0.15416667 -0.15 -0.14583333 -0.14166667 -0.1375 -0.13333333 -0.12916667 -0.125 -0.12083333 -0.11666667 -0.1125 -0.10833333 -0.10416667 -0.1 -0.09583333 -0.09166667 -0.0875 -0.08333333 -0.07916667 -0.075 -0.07083333 -0.06666667 -0.0625 -0.05833333 -0.05416667 -0.05 -0.04583333 -0.04166667 -0.0375 -0.03333333 -0.02916667 -0.025 -0.02083333 -0.01666667 -0.0125 -0.00833333 -0.00416667 0 0 0 0 0 0
  line L18 (7.333, 19.9984) -> (7.3326, 19.9973)
  line L19 (7.3326, 19.9973) -> (6.7131, 18.308)
  arc A10 (6.7131, 18.308) -> (4.2506, 19.0311) centre (0, 0) ccw
  line L20 (4.2506, 19.0311) -> (4.6428, 20.7871)
  line L21 (4.6428, 20.7871) -> (4.6431, 20.7882)
  spline S10 degree 5 poles (4.6431, 20.7882) (4.6431, 20.7884) (4.6432, 20.7887) (4.6433, 20.7892) (4.6434, 20.7899) (4.6437, 20.7911) (4.6439, 20.7924) (4.6442, 20.794) (4.6446, 20.7957) (4.6449, 20.7976) (4.6453, 20.7996) (4.6457, 20.8018) (4.6462, 20.8042) (4.6466, 20.8067) (4.6471, 20.8095) (4.6476, 20.8123) (4.6481, 20.8153) (4.6486, 20.8185) (4.6492, 20.8218) (4.6498, 20.8253) (4.6503, 20.8289) (4.6509, 20.8327) (4.6515, 20.8366) (4.6521, 20.8406) (4.6527, 20.8448) (4.6534, 20.8491) (4.654, 20.8536) (4.6546, 20.8582) (4.6553, 20.8629) (4.6559, 20.8677) (4.6566, 20.8727) (4.6573, 20.8778) (4.6579, 20.883) (4.6586, 20.8884) (4.6592, 20.8938) (4.6599, 20.8994) (4.6606, 20.9051) (4.6612, 20.911) (4.6619, 20.9169) (4.6625, 20.923) (4.6632, 20.9292) (4.6638, 20.9354) (4.6645, 20.9418) (4.6651, 20.9484) (4.6657, 20.955) (4.6664, 20.9617) (4.667, 20.9685) (4.6676, 20.9755) (4.6682, 20.9825) (4.6688, 20.9897) (4.6693, 20.9969) (4.6699, 21.0043) (4.6705, 21.0117) (4.671, 21.0193) (4.6716, 21.027) (4.6721, 21.0347) (4.6726, 21.0426) (4.6731, 21.0505) (4.6736, 21.0585) (4.6741, 21.0667) (4.6745, 21.0749) (4.675, 21.0832) (4.6754, 21.0916) (4.6758, 21.1002) (4.6762, 21.1087) (4.6766, 21.1174) (4.677, 21.1262) (4.6773, 21.1351) (4.6777, 21.144) (4.678, 21.1531) (4.6783, 21.1622) (4.6786, 21.1714) (4.6788, 21.1807) (4.6791, 21.1901) (4.6793, 21.1995) (4.6795, 21.2091) (4.6797, 21.2187) (4.6798, 21.2284) (4.68, 21.2382) (4.6801, 21.2481) (4.6802, 21.258) (4.6803, 21.268) (4.6803, 21.2781) (4.6804, 21.2883) (4.6804, 21.2986) (4.6804, 21.3089) (4.6804, 21.3193) (4.6803, 21.3298) (4.6802, 21.3404) (4.6801, 21.351) (4.68, 21.3617) (4.6798, 21.3725) (4.6797, 21.3833) (4.6795, 21.3943) (4.6792, 21.4053) (4.679, 21.4163) (4.6787, 21.4275) (4.6784, 21.4387) (4.6781, 21.45) (4.6777, 21.4613) (4.6773, 21.4727) (4.6769, 21.4842) (4.6765, 21.4958) (4.676, 21.5074) (4.6756, 21.5191) (4.675, 21.5308) (4.6745, 21.5426) (4.6739, 21.5545) (4.6733, 21.5664) (4.6727, 21.5785) (4.672, 21.5905) (4.6714, 21.6027) (4.6706, 21.6149) (4.6699, 21.6271) (4.6691, 21.6395) (4.6683, 21.6519) (4.6675, 21.6643) (4.6666, 21.6768) (4.6657, 21.6894) (4.6648, 21.702) (4.6639, 21.7147) (4.6629, 21.7275) (4.6619, 21.7403) (4.6608, 21.7531) (4.6598, 21.7661) (4.6587, 21.779) (4.6575, 21.7921) (4.6564, 21.8052) (4.6552, 21.8183) (4.6539, 21.8316) (4.6527, 21.8448) (4.6514, 21.8582) (4.65, 21.8715) (4.6487, 21.885) (4.6473, 21.8985) (4.6459, 21.912) (4.6444, 21.9256) (4.6429, 21.9392) (4.6414, 21.953) (4.6398, 21.9667) (4.6383, 21.9805) (4.6366, 21.9944) (4.635, 22.0083) (4.6333, 22.0223) (4.6316, 22.0363) (4.6298, 22.0503) (4.628, 22.0645) (4.6262, 22.0786) (4.6243, 22.0929) (4.6224, 22.1071) (4.6205, 22.1214) (4.6185, 22.1358) (4.6165, 22.1502) (4.6145, 22.1647) (4.6124, 22.1792) (4.6103, 22.1938) (4.6082, 22.2084) (4.606, 22.223) (4.6038, 22.2377) (4.6016, 22.2525) (4.5993, 22.2673) (4.597, 22.2821) (4.5946, 22.297) (4.5922, 22.3119) (4.5898, 22.3269) (4.5873, 22.3419) (4.5848, 22.357) (4.5823, 22.3721) (4.5797, 22.3873) (4.5771, 22.4025) (4.5745, 22.4177) (4.5718, 22.433) (4.5691, 22.4484) (4.5663, 22.4637) (4.5636, 22.4792) (4.5607, 22.4946) (4.5579, 22.5101) (4.555, 22.5257) (4.552, 22.5412) (4.549, 22.5569) (4.546, 22.5725) (4.543, 22.5883) (4.5399, 22.604) (4.5368, 22.6198) (4.5336, 22.6356) (4.5304, 22.6515) (4.5272, 22.6674) (4.5239, 22.6834) (4.5206, 22.6993) (4.5172, 22.7154) (4.5138, 22.7314) (4.5104, 22.7475) (4.5069, 22.7637) (4.5034, 22.7799) (4.4998, 22.7961) (4.4963, 22.8124) (4.4926, 22.8286) (4.489, 22.845) (4.4853, 22.8613) (4.4815, 22.8777) (4.4777, 22.8942) (4.4739, 22.9107) (4.4701, 22.9272) (4.4662, 22.9437) (4.4622, 22.9603) (4.4582, 22.9769) (4.4542, 22.9936) (4.4502, 23.0103) (4.4461, 23.027) (4.4419, 23.0438) (4.4378, 23.0606) (4.4335, 23.0774) (4.4293, 23.0942) (4.425, 23.1111) (4.4206, 23.1281) (4.4163, 23.145) (4.4119, 23.162) (4.4074, 23.179) (4.4029, 23.1961) (4.3984, 23.2132) (4.3938, 23.2303) (4.3892, 23.2475) (4.3845, 23.2647) (4.3798, 23.2819) (4.3751, 23.2991) (4.3703, 23.3164) (4.3655, 23.3337) (4.3606, 23.3511) (4.3557, 23.3684) (4.3508, 23.3858) (4.3458, 23.4033) (4.3408, 23.4207) (4.3357, 23.4382) (4.3306, 23.4558) (4.3255, 23.4733) (4.3203, 23.4909) (4.315, 23.5085) (4.3098, 23.5261) (4.3045, 23.5438) (4.2991, 23.5615) (4.2937, 23.5792) (4.2894, 23.5934) (4.2861, 23.6041) (4.2839, 23.6112) (4.2828, 23.6148) knots 0 0 0 0 0 0 0.00416667 0.00833333 0.0125 0.01666667 0.02083333 0.025 0.02916667 0.03333333 0.0375 0.04166667 0.04583333 0.05 0.05416667 0.05833333 0.0625 0.06666667 0.07083333 0.075 0.07916667 0.08333333 0.0875 0.09166667 0.09583333 0.1 0.10416667 0.10833333 0.1125 0.11666667 0.12083333 0.125 0.12916667 0.13333333 0.1375 0.14166667 0.14583333 0.15 0.15416667 0.15833333 0.1625 0.16666667 0.17083333 0.175 0.17916667 0.18333333 0.1875 0.19166667 0.19583333 0.2 0.20416667 0.20833333 0.2125 0.21666667 0.22083333 0.225 0.22916667 0.23333333 0.2375 0.24166667 0.24583333 0.25 0.25416667 0.25833333 0.2625 0.26666667 0.27083333 0.275 0.27916667 0.28333333 0.2875 0.29166667 0.29583333 0.3 0.30416667 0.30833333 0.3125 0.31666667 0.32083333 0.325 0.32916667 0.33333333 0.3375 0.34166667 0.34583333 0.35 0.35416667 0.35833333 0.3625 0.36666667 0.37083333 0.375 0.37916667 0.38333333 0.3875 0.39166667 0.39583333 0.4 0.40416667 0.40833333 0.4125 0.41666667 0.42083333 0.425 0.42916667 0.43333333 0.4375 0.44166667 0.44583333 0.45 0.45416667 0.45833333 0.4625 0.46666667 0.47083333 0.475 0.47916667 0.48333333 0.4875 0.49166667 0.49583333 0.5 0.50416667 0.50833333 0.5125 0.51666667 0.52083333 0.525 0.52916667 0.53333333 0.5375 0.54166667 0.54583333 0.55 0.55416667 0.55833333 0.5625 0.56666667 0.57083333 0.575 0.57916667 0.58333333 0.5875 0.59166667 0.59583333 0.6 0.60416667 0.60833333 0.6125 0.61666667 0.62083333 0.625 0.62916667 0.63333333 0.6375 0.64166667 0.64583333 0.65 0.65416667 0.65833333 0.6625 0.66666667 0.67083333 0.675 0.67916667 0.68333333 0.6875 0.69166667 0.69583333 0.7 0.70416667 0.70833333 0.7125 0.71666667 0.72083333 0.725 0.72916667 0.73333333 0.7375 0.74166667 0.74583333 0.75 0.75416667 0.75833333 0.7625 0.76666667 0.77083333 0.775 0.77916667 0.78333333 0.7875 0.79166667 0.79583333 0.8 0.80416667 0.80833333 0.8125 0.81666667 0.82083333 0.825 0.82916667 0.83333333 0.8375 0.84166667 0.84583333 0.85 0.85416667 0.85833333 0.8625 0.86666667 0.87083333 0.875 0.87916667 0.88333333 0.8875 0.89166667 0.89583333 0.9 0.90416667 0.90833333 0.9125 0.91666667 0.92083333 0.925 0.92916667 0.93333333 0.9375 0.94166667 0.94583333 0.95 0.95416667 0.95833333 0.9625 0.96666667 0.97083333 0.975 0.97916667 0.98333333 0.9875 0.99166667 0.99583333 1 1 1 1 1 1
  arc A11 (4.2828, 23.6148) -> (2.5437, 23.8648) centre (0, 0) ccw